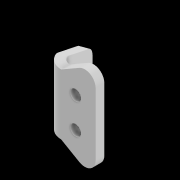
# Autodesk Inventor part: ChestPelvisConnector
Saved by Autodesk Inventor 2020 (Build 240168000, 168)
## iProperties
Created: 2020-05-07
Part Number: ChestPelvisConnector
Material: Generic
Document SubType Name: Sheet Metal
Designer: valer
Density: 1 g/cm^3
Sheet Metal Rule: Default
Appearance: Default
Author: valer
Autodesk Inventor part; units mm, degrees
note: some values were not read from the file. Chosen so that the rebuilt part matches the saved one: flange form of "Plate2".
ref_plane "YZ Plane" through (0, 0, 0) normal (1, 0, 0) x (0, 1, 0)
ref_plane "XZ Plane" through (0, 0, 0) normal (0, 1, 0) x (-1, 0, 0)
ref_plane "XY Plane" through (0, 0, 0) normal (0, 0, 1) x (1, 0, 0)
sketch "Base" plane through (0, 0, 0) normal (0, 0, 1) x (1, 0, 0)
  line L0 (-23.4822, 45.3385) -> (0, 58.896)
  line L1 (-23.4822, 13.5575) -> (-23.4822, 45.3385)
  line L2 (0, 0) -> (-23.4822, 13.5575)
  line L3 (0, 58.896) -> (0, 0)
  circle A0 centre (-11.7411, 38.3467) radius 3.175
  circle A1 centre (-11.7411, 20.5493) radius 3.175
  line L4 (-11.7411, 38.3467) -> (-11.7411, 20.5493) construction
  line L5 (-11.7411, 29.448) -> (-23.4822, 29.448) construction
  line L6 (-20.2078, 47.229) -> (-20.2078, 11.667)
  dimension "d0" = 58.896
  dimension "d1" = 27.1149
  dimension "d2" = 60
  dimension "d3" = 60
  dimension "d4" = 31.7811
  dimension "d5" = 6.35
  dimension "d6" = 17.7974
  dimension "d7" = 11.7411
  dimension "d8" = 11.7411
  dimension "d9" = 8.4667
  measures "d0" distance of L2.start L0.end
  measures "d1" distance of L2.start L1.start
  measures "d2" angle of L3 L2
  measures "d3" angle of L3 L0
  measures "d4" distance of L1.start L0.start
  measures "d5" diameter of A1
  measures "d6" distance of L4.start L4.end
  measures "d7" distance between parallel lines of L3 L4
  measures "d8" distance of L5.start L5.end
  measures "d9" distance between parallel lines of L4 L6
extrude "Plate1" add sketch "Base" along normal blind 5.08 contours L0 L3 L2 L6
sketch "Sketch2" plane through (-24.9814, 47.229, -3.3425) normal (-0.9396926, 0, 0.3420201) x (0, -1, 0)
  line L0 (35.562, 0) -> (0, 0)
  line L1 (0, 0) -> (0, -24.6359)
  line L2 (0, -24.6359) -> (35.562, -24.6359)
  line L3 (35.562, -24.6359) -> (35.562, 0)
  constraints: 6 end point, 1 horizontal, 1 perpendicular, 1 vertical
edge flange "ShockFlangeFeature" height 31.75 angle 70 thickness 5.08 bend radius 5.08 thickness toward (-0.9396926, 0, 0.3420201) relief tear relief width 5.08 relief depth 2.54 edges at (-20.2078, 29.448, 0) wall of the first edge with corners at (-24.9814, 11.667, -3.3425) (-24.9814, 47.229, -3.3425) (-33.4074, 47.229, -26.4927) (-33.4074, 11.667, -26.4927)
bend "Bend1"
corner "Corner1"
sketch "ShockFlangeDraft" plane through (-33.4074, 11.667, -26.4927) normal (0.9396926, 0, -0.3420201) x (-0.3420201, 0, -0.9396926)
  line L0 (-24.6359, 35.562) -> (-24.6359, 0) projected
  line L1 (0, 0) -> (-24.6359, 0) projected
  line L2 (0, 0) -> (0, 35.562) projected
  line L3 (0, 35.562) -> (-24.6359, 35.562) projected
  line L4 (-24.2986, 35.562) -> (0, 24.2098)
  line L5 (-24.6359, 0) -> (0, 11.5098)
  line L6 (0, 17.781) -> (-24.6359, 17.781) construction
  line L7 (-24.6359, 35.562) -> (-24.6359, 0) projected
  point P0 (-36.321, -11.667)
  dimension "d34" = 64.958
  dimension "d35" = 64.958
  dimension "d36" = 12.7
  constraints: 6 end point, 3 point on line, 2 midpoint
  measures "d34" angle of L4 L0
  measures "d35" angle of L5 L0
  measures "d36" distance of L5.end L4.end
extrude "ShockFlangeDraftFeature" cut sketch "ShockFlangeDraft" against normal blind 25.4 contours L5 L2 L1 | L3 L2 L4
fillet "FilletsFeature" radius 6.35 6 edges at (-35.7942, 35.8768, -25.624) (0, 58.896, 2.54) (0, 0, 2.54) (-27.4836, 47.229, -2.7907) (-35.7942, 23.1768, -25.624) (-27.3682, 11.667, -2.4738)
sketch "ShockMountHole" plane through (-29.755, 11.667, -1.6051) normal (-0.9396926, 0, 0.3420201) x (0.3420201, 0, 0.9396926)
  circle A0 centre (-14.6604, 17.8598) radius 9.9755 construction
  line L0 (-24.6359, 15.5519) -> (-24.6359, 20.1677) projected
  line L1 (-20.9737, 25.9208) -> (-1.6149, 34.9651) projected
  line L2 (-1.2776, 0.5969) -> (-20.9737, 9.7989) projected
  circle A1 centre (-14.6604, 17.8598) radius 3.175
  point P0 (-0.1927, 28.9261)
  dimension "d37" = 6.35
  constraints: 3 tangent, 2 centre point, 1 coincident
  measures "d37" diameter of A1
hole "ShockMountHoleFeature" at (-34.7692, 29.5268, -15.3813) direction (0.9396926, 0, -0.3420201) diameter 6.35 end through all
equation "\"d35\" = d34"
equation "\"d32\" = Thickness"
equation "\"d10\" = Thickness"
equation "\"d11\" = BendReliefWidth"
equation "\"d12\" = BendReliefDepth"
equation "\"d13\" = MinimumRemnant"
equation "\"d14\" = TransitionRadius"
equation "\"d17\" = BendRadius"
equation "\"d18\" = CornerReliefSize"
equation "\"d19\" = GapSize"
equation "\"d20\" = JacobiRadiusSize"
equation "\"BendRadius\" = Thickness"
equation "\"BendReliefWidth\" = Thickness"
equation "\"BendReliefDepth\" = 0.5 * Thickness"
equation "\"CornerReliefSize\" = 4 * Thickness"
equation "\"MinimumRemnant\" = 2 * Thickness"
equation "\"TransitionRadius\" = BendRadius"
equation "\"JacobiRadiusSize\" = BendRadius"
equation "\"GapSize\" = Thickness"
equation "\"Thickness\" = 5.08"
body "Solid1"
